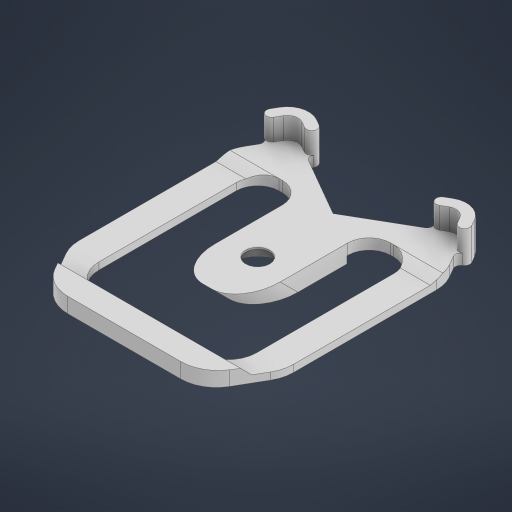
# Autodesk Inventor part: LilypadClipCutout
Saved by Autodesk Inventor 2023 (Build 270158000, 158)
## iProperties
Created: 2022-07-22
Part Number: LilypadClipCutout
Material: Generic
Document SubType Name: Modeling
Designer: jevan
Density: 1 g/cm^3
Appearance: Default
Author: jevan
Autodesk Inventor part; units mm, degrees
ref_plane "YZ Plane" through (0, 0, 0) normal (1, 0, 0) x (0, 1, 0)
ref_plane "XZ Plane" through (0, 0, 0) normal (0, 1, 0) x (-1, 0, 0)
ref_plane "XY Plane" through (0, 0, 0) normal (0, 0, 1) x (1, 0, 0)
sketch "Sketch1" plane through (0, 0, 0) normal (0, 0, 1) x (1, 0, 0)
  line L0 (-27.3013, -27.7128) -> (-40.4145, -5)
  line L1 (-40.4145, 5) -> (-24.5374, 32.5)
  line L2 (-15.8771, 37.5) -> (15.8771, 37.5)
  line L3 (24.5374, 32.5) -> (40.4145, 5)
  line L4 (40.4145, -5) -> (27.3013, -27.7128)
  line L5 (21.6506, -37.5) -> (-21.6506, -37.5)
  line L6 (16.3731, -30.641) -> (0, -21.188)
  line L7 (0, -21.188) -> (-16.3731, -30.641)
  circle A0 centre (0, 0) radius 4.75
  line L8 (43.3013, 0) -> (41.7543, 0)
  arc A1 (20.7032, -33.141) -> (24.8013, -32.0429) centre (22.2032, -30.5429) ccw
  arc A2 (-24.8013, -32.0429) -> (-20.7032, -33.141) centre (-22.2032, -30.5429) ccw
  arc A3 (40.4145, -5) -> (40.4145, 5) centre (31.7543, 0) ccw
  arc A4 (24.5374, 32.5) -> (15.8771, 37.5) centre (15.8771, 27.5) ccw
  arc A5 (-15.8771, 37.5) -> (-24.5374, 32.5) centre (-15.8771, 27.5) ccw
  arc A6 (-40.4145, 5) -> (-40.4145, -5) centre (-31.7543, 0) ccw
  circle A7 centre (0, 0) radius 3.375
  line L9 (0, -21.188) -> (0, -37.5)
  circle A8 centre (0, 0) radius 7.225
  line L10 (0, 0) -> (-7.225, 0)
  line L11 (-9.225, 0) -> (-9.225, -16.1218)
  line L12 (-19.2032, -35.7391) -> (0, -24.6521)
  line L13 (0, -24.6521) -> (19.2032, -35.7391)
  arc A9 (19.2032, -35.7391) -> (27.3993, -33.5429) centre (22.2032, -30.5429) ccw
  line L14 (27.3993, -33.5429) -> (43.0126, -6.5)
  arc A10 (43.0126, -6.5) -> (43.0126, 6.5) centre (31.7543, 0) ccw
  line L15 (43.0126, 6.5) -> (27.1355, 34)
  arc A11 (27.1355, 34) -> (15.8771, 40.5) centre (15.8771, 27.5) ccw
  line L16 (15.8771, 40.5) -> (-15.8771, 40.5)
  arc A12 (-15.8771, 40.5) -> (-27.1355, 34) centre (-15.8771, 27.5) ccw
  line L17 (-27.1355, 34) -> (-43.0126, 6.5)
  arc A13 (-43.0126, 6.5) -> (-43.0126, -6.5) centre (-31.7543, 0) ccw
  line L18 (-43.0126, -6.5) -> (-27.3993, -33.5429)
  arc A14 (-27.3993, -33.5429) -> (-19.2032, -35.7391) centre (-22.2032, -30.5429) ccw
  line L19 (-15.225, -22.1218) -> (-16.1451, -22.1218)
  line L20 (-22.1451, -16.1218) -> (-22.1451, 22.5)
  line L21 (-14.1451, 30.5) -> (0, 30.5)
  arc A15 (-14.1451, 30.5) -> (-22.1451, 22.5) centre (-14.1451, 22.5) ccw
  arc A16 (-22.1451, -16.1218) -> (-16.1451, -22.1218) centre (-16.1451, -16.1218) ccw
  arc A17 (-15.225, -22.1218) -> (-9.225, -16.1218) centre (-15.225, -16.1218) ccw
  line L22 (0, 0) -> (0, 30.5)
  line L23 (9.225, 0) -> (9.225, -16.1218)
  line L24 (15.225, -22.1218) -> (16.1451, -22.1218)
  line L25 (22.1451, -16.1218) -> (22.1451, 22.5)
  line L26 (14.1451, 30.5) -> (0, 30.5)
  arc A18 (22.1451, 22.5) -> (14.1451, 30.5) centre (14.1451, 22.5) ccw
  arc A19 (16.1451, -22.1218) -> (22.1451, -16.1218) centre (16.1451, -16.1218) ccw
  arc A20 (9.225, -16.1218) -> (15.225, -22.1218) centre (15.225, -16.1218) ccw
  circle A21 centre (0, 0) radius 9.225
  line L27 (-22.2032, -30.5429) -> (-24.8013, -32.0429)
  line L28 (-22.2032, -30.5429) -> (-20.7032, -33.141)
  line L29 (22.2032, -30.5429) -> (20.7032, -33.141)
  line L30 (22.2032, -30.5429) -> (24.8013, -32.0429)
  arc A22 (-25.8013, -30.3109) -> (-28.3993, -31.8109) centre (-27.1003, -31.0609) ccw
  arc A23 (-17.4711, -34.7391) -> (-18.9711, -32.141) centre (-18.2211, -33.4401) ccw
  arc A24 (28.3993, -31.8109) -> (25.8013, -30.3109) centre (27.1003, -31.0609) ccw
  arc A25 (18.9711, -32.141) -> (17.4711, -34.7391) centre (18.2211, -33.4401) ccw
  line L31 (-14.1451, 30.5) -> (-25.6921, 30.5)
  line L32 (14.1451, 30.5) -> (25.6921, 30.5)
  line L33 (-16.1451, -22.1218) -> (-30.5293, -22.1218)
  line L34 (16.1451, -22.1218) -> (30.5293, -22.1218)
  line L35 (24.8013, -32.0429) -> (40.4145, -5)
  arc A26 (40.4145, -5) -> (40.4145, 5) centre (31.7543, 0) ccw
  line L36 (40.4145, 5) -> (24.5374, 32.5)
  arc A27 (24.5374, 32.5) -> (15.8771, 37.5) centre (15.8771, 27.5) ccw
  line L37 (15.8771, 37.5) -> (-15.8771, 37.5)
  arc A28 (-15.8771, 37.5) -> (-24.5374, 32.5) centre (-15.8771, 27.5) ccw
  line L38 (-24.5374, 32.5) -> (-40.4145, 5)
  arc A29 (-40.4145, 5) -> (-40.4145, -5) centre (-31.7543, 0) ccw
  line L39 (-40.4145, -5) -> (-24.8013, -32.0429)
  arc A30 (20.7032, -33.141) -> (24.8013, -32.0429) centre (22.2032, -30.5429) ccw
  line L40 (20.7032, -33.141) -> (0, -21.188)
  line L41 (0, -21.188) -> (-20.7032, -33.141)
  arc A31 (-24.8013, -32.0429) -> (-20.7032, -33.141) centre (-22.2032, -30.5429) ccw
  line L42 (27.8503, -29.7619) -> (27.8503, -29.7619)
  line L43 (16.9221, -32.6901) -> (16.9221, -32.6901)
  line L44 (-16.9221, -32.6901) -> (-16.9221, -32.6901)
  line L45 (-27.8503, -29.7619) -> (-27.8503, -29.7619)
  arc A32 (27.3013, -27.7128) -> (27.8503, -29.7619) centre (28.6003, -28.4628) ccw
  arc A33 (16.9221, -32.6901) -> (16.3731, -30.641) centre (15.6231, -31.9401) ccw
  arc A34 (-16.3731, -30.641) -> (-16.9221, -32.6901) centre (-15.6231, -31.9401) ccw
  arc A35 (-27.8503, -29.7619) -> (-27.3013, -27.7128) centre (-28.6003, -28.4628) ccw
  line L46 (-24.5374, 32.5) -> (-21.6506, 37.5)
  line L47 (-15.8771, 37.5) -> (-21.6506, 37.5)
  line L48 (15.8771, 37.5) -> (21.6506, 37.5)
  line L49 (24.5374, 32.5) -> (21.6506, 37.5)
  line L50 (30.1451, -22.7872) -> (30.1451, 22.7872)
  line L51 (-30.1451, -22.7872) -> (-30.1451, 22.7872)
  point P0 (-43.3013, 0)
  point P1 (36.8061, -2.25)
  point P2 (6.0982, -2.25)
  point P3 (19.9965, -30.1349)
  point P4 (4.9976, -4.1562)
  point P5 (-6.0982, 2.25)
  point P6 (-36.8061, 2.25)
  point P7 (-36.8061, -2.25)
  point P8 (-6.0982, -2.25)
  point P9 (-20.3516, 30.75)
  point P10 (-4.9976, 4.1562)
  point P11 (-1.1005, 6.4062)
  point P12 (-16.4545, 33)
  point P13 (16.4545, 33)
  point P14 (1.1005, 6.4062)
  point P15 (4.9976, 4.1562)
  point P16 (20.3516, 30.75)
  point P17 (36.8061, 2.25)
  point P18 (6.0982, 2.25)
  point P19 (1.1005, -6.4062)
  point P20 (12.2023, -25.6349)
  point P21 (-4.9976, -4.1562)
  point P22 (-19.9965, -30.1349)
  point P23 (-12.2023, -25.6349)
  point P24 (-1.1005, -6.4062)
  point P25 (-9.225, -26.5141)
  point P26 (7, 0)
  point P27 (0, 7.225)
  point P28 (17.4711, -34.7391)
  point P29 (28.3993, -31.8109)
  point P30 (25.8013, -30.3109)
  point P31 (24.8013, -32.0429)
  point P32 (20.7032, -33.141)
  point P33 (18.9711, -32.141)
  point P34 (-20.7032, -33.141)
  point P35 (-24.8013, -32.0429)
  point P36 (30.1451, -22.1218)
  point P37 (30.1451, 22.7872)
  point P38 (-30.1451, 22.7872)
  point P39 (-30.1451, -22.1218)
  point P40 (-27.8503, -29.7619)
  point P41 (-16.9221, -32.6901)
  point P42 (27.8503, -29.7619)
  dimension "d28" = 14.45
  dimension "d1" = 9.5
  dimension "d3" = 120
  dimension "d6" = 75
  dimension "d17" = 40
  dimension "d18" = 3
  dimension "d19" = 10
  dimension "d22" = 6.75
  dimension "d24" = 3
  dimension "d25" = 8
  dimension "d26" = 6
  dimension "d27" = 6
  dimension "d29" = 2
  dimension "d30" = 2
  dimension "d31" = 2
  dimension "d36" = 6
  dimension "d37" = 0
  dimension "d38" = 0
  dimension "d39" = 0
  dimension "d40" = 0
  dimension "d41" = 0
  dimension "d42" = 1.5
  dimension "d45" = 7
  dimension "d66" = 8
  constraints: 104 end point, 71 point on circle, 35 centre point, 35 tangent, 30 point on line, 17 symmetric about line, 11 perpendicular, 8 equal radius, 4 coincident, 4 vertical, 3 horizontal, 2 collinear, 1 concentric, 1 midpoint, 1 parallel, 36 other
  measures "d1" diameter of A0
  measures "d3" angle of L7 L6
  measures "d6" distance between parallel lines of L5 L2
  measures "d17" distance from line of L8.start L6
  measures "d18" radius of A1
  measures "d19" radius of A3
  measures "d22" diameter of A7
  measures "d24" distance between parallel lines of L7 L12
  measures "d25" radius of A15
  measures "d26" radius of A16
  measures "d27" distance edge to line of A17 L7
  measures "d30" distance from line of A22.centre L27
  measures "d31" distance from line of L28 A23.centre
  measures "d36" distance edge to line of A15 L1
  measures "d37" distance between parallel lines of L4 L35
  measures "d38" radial gap between concentric circles of A1 A30
  measures "d39" distance between parallel lines of L6 L40
  measures "d40" distance between parallel lines of L7 L41
  measures "d41" radial gap between concentric circles of A2 A31
  measures "d42" radius of A32
  measures "d45" distance between parallel lines of L2 L26
  measures "d66" distance between parallel lines of L25 L50
extrude "Extrusion1" add sketch "Sketch1" along normal blind 5 contours L0 L51 L33 L19 A17 L11 A21 L23 A20 L24 L34 L50 L4 L35 L30 L29 L40 L6 L7 L41 L28 L27 L39 | L39 A22 A35 | L39 A2 L41 A23 L12 A14 L18 A22 | L51 L1 L31 A15 L20 A16 L33 | L27 L28 A2 | L1 A5 L2 A4 L3 L32 L26 L21 L31 | L41 A34 A23 | A21 | L32 L3 L50 L34 A19 L25 A18 | L40 A25 A33 | A25 L40 A1 L35 A24 L14 A9 L13 | L29 L30 A1 | L35 A32 A24
extrude "Extrusion2" add sketch "Sketch1" along normal blind 0.5 contours A0 L10 A7 L22 | A0 L22 A8 L10 | L22 A7 L10 A0 | A0 L10 A8 L22
extrude "Extrusion3" cut sketch "Sketch1" along normal blind 1 contours L0 A6 L1 L51 L33 | L51 L1 L31 A15 L20 A16 L33 | L32 L3 L50 L34 A19 L25 A18 | L3 A3 L4 L34 L50
extrude "Extrusion4" add sketch "Sketch1" against normal blind 6 contours L39 A2 L41 A23 L12 A14 L18 A22 | A25 L40 A1 L35 A24 L14 A9 L13
extrude "Extrusion5" add sketch "Sketch1" against normal blind 1.25 contours L1 A5 L2 A4 L3 L32 L26 L21 L31
chamfer "Chamfer1" distance 7 distance2 0.25 1 edges at (0, 30.5, -1.25) measured on face at (0, 31, -1.25)
chamfer "Chamfer2" distance 1 angle 75 1 edges at (-23.1451, -22.1218, 1) measured on face at (-23.1451, -22.1218, 0.5)
chamfer "Chamfer3" distance 1 angle 75 1 edges at (23.1451, -22.1218, 1) measured on face at (23.1451, -22.1218, 0.5)
sketch "Sketch2" plane through (0, 0, 0) normal (0, 0, -1) x (-1, 0, 0)
  line L0 (9.225, 0) -> (9.225, -16.1218) projected
  line L1 (9.225, 0) -> (-9.225, 0)
  line L2 (-9.225, 0) -> (-9.225, 9.225)
  line L3 (-9.225, 9.225) -> (9.225, 9.225)
  line L4 (9.225, 9.225) -> (9.225, 0)
  circle A0 centre (0, 0) radius 9.225
  arc A1 (9.225, 0) -> (-9.225, 0) centre (0, 0) ccw projected
  point P0 (0, 9.225)
  constraints: 8 end point, 2 parallel, 1 centre point, 1 coincident, 1 horizontal, 1 perpendicular, 1 tangent
fillet "Fillet3" radius 10 4 edges at (-30.1451, -22.7872, 2.5) (-30.1451, 22.7872, 3) (30.1451, -22.7872, 2.5) (30.1451, 22.7872, 3)
extrude "Extrusion7" add sketch "Sketch2" against normal up to surface (5 mm away) contours A0 L3 L4 | L2 L3 A0
draft "FaceDraft3" angle 45 pull direction (0, 0, 1) faces at (-3.075, 9.225, 1.6667) fixed edges at (0, 9.225, 5)
fillet "Fillet10" radius 8 2 edges at (9.225, 11.725, 2.5) (-9.225, 11.725, 2.5)
chamfer "Chamfer8" distance 2 angle 45 2 edges at (19.9186, 30.5, 1) (-19.9186, 30.5, 1)
sketch "Sketch7" plane through (0, 0, 5) normal (0, 0, 1) x (1, 0, 0)
  line L0 (0, -21.188) -> (16.3731, -30.641) projected
  line L1 (0, -21.188) -> (-9.225, -15.862)
  line L2 (-9.225, -16.1218) -> (-9.225, -2.0887) projected
  line L3 (0, -21.188) -> (0, -36.5429)
  line L4 (0, -36.5429) -> (-30.1451, -36.5429)
  line L5 (-30.1451, -36.5429) -> (-30.1451, 37.5)
  line L6 (-30.1451, 37.5) -> (0, 37.5)
  line L7 (0, -21.188) -> (9.225, -15.862)
  line L8 (0, -36.5429) -> (30.1451, -36.5429)
  line L9 (30.1451, -36.5429) -> (30.1451, 37.5)
  line L10 (30.1451, 37.5) -> (0, 37.5)
  line L11 (-30.1451, 20.1077) -> (-30.1451, -20.1077) projected
  arc A0 (-27.3993, -33.5429) -> (-19.2032, -35.7391) centre (-22.2032, -30.5429) ccw projected
  line L12 (15.8771, 37.5) -> (-15.8771, 37.5) projected
  line L13 (-9.225, -15.862) -> (-9.225, 14.225)
  line L14 (-9.225, 14.225) -> (0, 14.225)
  line L15 (-1.225, 14.225) -> (1.225, 14.225) projected
  line L16 (9.225, -15.862) -> (9.225, 14.225)
  line L17 (9.225, 14.225) -> (0, 14.225)
  line L18 (9.225, -15.862) -> (-9.225, -15.862)
  point P0 (0, 0)
  point P1 (-9.225, -2.0887)
  constraints: 28 end point, 5 perpendicular, 4 collinear, 4 symmetric about line, 3 point on line, 1 tangent, 1 vertical
extrude "Extrusion10" cut sketch "Sketch7" against normal blind 2 contours L1 L18 L7 | L4 L5 L6 L10 L9 L8
body "Solid1"
